Autodesk Fusion 360 part; units mm, degrees
(part 2 of 2)
sketch "Sketch5" plane through (0, 0, 3) normal (0, 0, 1) x (-1, 0, 0)
  circle A0 centre (19.806368, 49.24591) radius 1.5
  circle A1 centre (-47.207036, 20.58349) radius 1.5
  circle A2 centre (47.000001, -22) radius 1.5
  circle A3 centre (-21.042031, -45.95674) radius 1.5
  arc A4 (55, 15) -> (15, 55) centre (15, 15) ccw
  line L0 (15, 55) -> (-15, 55)
  arc A5 (-15, 55) -> (-55, 15) centre (-15, 15) ccw
  line L1 (-55, 15) -> (-55, -15)
  arc A6 (-55, -15) -> (-15, -55) centre (-15, -15) ccw
  line L2 (-15, -55) -> (15, -55)
  arc A7 (15, -55) -> (55, -15) centre (15, -15) ccw
  line L3 (55, -15) -> (55, 15)
  spline S0 degree 3 poles (33.028609, 28.071836) (33.020542, 28.201801) (33.037938, 28.332099) (33.121694, 28.578692) (33.187255, 28.69263) (33.35836, 28.888963) (33.462269, 28.969481) (33.695102, 29.086154) (33.821799, 29.121194) (34.01862, 29.136006) (34.085931, 29.134286) (34.219188, 29.117378) (34.284796, 29.102233) (34.348388, 29.080627) knots 0 0 0 0 0.03906445 0.03906445 0.07812889 0.07812889 0.11719334 0.11719334 0.15625779 0.15625779 0.17640658 0.17640658 0.19655538 0.19655538 0.19655538 0.19655538
  spline S1 degree 3 poles (33.028609, 28.071836) (33.070325, 27.399743) (33.167612, 26.697689) (33.534795, 25.632572) (33.720748, 25.326789) (34.102443, 24.870238) (34.323648, 24.704363) (34.841834, 24.437201) (35.152732, 24.346965) (36.444281, 24.071142) (37.766512, 23.970732) (40.258569, 22.861355) (41.159058, 22.248794) (42.580431, 20.763821) (43.105542, 19.944649) (43.820617, 18.088798) (43.981774, 17.098841) (44.002724, 14.699008) (43.726283, 13.299817) (42.523118, 9.293833) (41.144668, 6.638018) (39.093015, 2.019583) (38.33328, 0.102917) (37.445131, -3.451458) (37.219765, -4.824183) (37.092807, -6.21584) knots 0.12920252 0.12920252 0.12920252 0.12920252 0.29400635 0.29400635 0.41743504 0.41743504 0.55008159 0.55008159 0.70447822 0.70447822 1.12919382 1.12919382 1.40886872 1.40886872 1.66213987 1.66213987 1.92272299 1.92272299 2.28120027 2.28120027 3.00174739 3.00174739 3.49260172 3.49260172 3.80923678 3.80923678 3.80923678 3.80923678
  spline S2 degree 3 poles (38.088834, -7.30669) (37.958619, -7.306711) (37.829645, -7.281298) (37.588698, -7.182465) (37.479028, -7.10999) (37.293642, -6.927081) (37.219699, -6.818395) (37.13638, -6.622803) (37.113583, -6.543309) (37.088005, -6.380538) (37.085323, -6.297883) (37.092807, -6.21584) knots 0 0 0 0 0.03906445 0.03906445 0.07812889 0.07812889 0.11719334 0.11719334 0.14190861 0.14190861 0.16662387 0.16662387 0.16662387 0.16662387
  line L4 (38.088834, -7.30669) -> (44.477012, 2.623123)
  arc A8 (49.249836, -0.9845) -> (44.477012, 2.623123) centre (47.000001, 1) ccw
  line L5 (49.249836, -0.9845) -> (41.439374, -9.839254)
  line L6 (41.439374, -9.839254) -> (37.553028, -14.980826)
  spline S3 degree 3 poles (37.355491, -15.680812) (37.343423, -15.556976) (37.354571, -15.431969) (37.422156, -15.192477) (37.478002, -15.080084) (37.553028, -14.980826) knots 0 0 0 0 0.03732672 0.03732672 0.07465345 0.07465345 0.07465345 0.07465345
  spline S4 degree 3 poles (37.355491, -15.680812) (37.717512, -19.395606) (38.115975, -22.808309) (37.32032, -26.055888) (37.037048, -26.721878) (36.287107, -27.771965) (35.864089, -28.165019) (34.777138, -28.862662) (34.111926, -29.125105) (33.399815, -29.330821) knots 0.03917141 0.03917141 0.03917141 0.03917141 1.16482767 1.16482767 1.51694644 1.51694644 1.81940977 1.81940977 2.17139083 2.17139083 2.17139083 2.17139083
  spline S5 degree 3 poles (32.689476, -30.136274) (32.709693, -30.007638) (32.754843, -29.884181) (32.889924, -29.661523) (32.978563, -29.56445) (33.178711, -29.416652) (33.285884, -29.363733) (33.399815, -29.330821) knots 0 0 0 0 0.03906445 0.03906445 0.07812889 0.07812889 0.11370578 0.11370578 0.11370578 0.11370578
  line L7 (32.689476, -30.136274) -> (31.798898, -35.802654)
  line L8 (31.798898, -35.802654) -> (29.963534, -47.466334)
  arc A9 (24.140467, -46.09277) -> (29.963534, -47.466334) centre (27, -47.000001) ccw
  line L9 (24.140467, -46.09277) -> (27.711083, -34.838407)
  line L10 (27.711083, -34.838407) -> (28.342134, -32.16314)
  spline S6 degree 3 poles (26.916548, -31.04169) (27.032682, -30.982795) (27.15921, -30.947146) (27.418808, -30.926354) (27.549397, -30.94141) (27.797453, -31.020732) (27.912548, -31.084239) (28.111917, -31.251796) (28.194285, -31.354245) (28.310066, -31.575309) (28.346065, -31.690083) (28.375918, -31.926876) (28.369531, -32.046994) (28.342134, -32.16314) knots 0 0 0 0 0.03906445 0.03906445 0.07812889 0.07812889 0.11719334 0.11719334 0.15625779 0.15625779 0.1920579 0.1920579 0.227858 0.227858 0.227858 0.227858
  spline S7 degree 3 poles (26.916548, -31.04169) (26.501678, -31.252085) (26.107211, -31.499509) (24.939768, -32.410184) (24.29803, -33.165919) (22.091994, -36.254574) (20.565282, -39.28296) (15.831093, -43.406948) (14.024745, -44.411258) (11.181859, -45.397232) (9.989834, -45.607) (8.140393, -45.536834) (7.398883, -45.389219) (6.139798, -44.814776) (5.640001, -44.453149) (4.7208, -43.481488) (4.349579, -42.883055) (3.462916, -41.050115) (3.101277, -39.69498) (2.31369, -37.647221) (1.945545, -36.882494) (1.036613, -35.79784) (0.593737, -35.439307) (-0.469029, -34.890024) (-1.078331, -34.709667) (-2.902765, -34.442063) (-4.21808, -34.494421) (-5.659673, -34.662249) knots 0.20837114 0.20837114 0.20837114 0.20837114 0.35937386 0.35937386 0.67047774 0.67047774 1.4465987 1.4465987 1.89541729 1.89541729 2.22492207 2.22492207 2.45047306 2.45047306 2.6397202 2.6397202 2.85015814 2.85015814 3.24794097 3.24794097 3.51947787 3.51947787 3.71561689 3.71561689 3.91564309 3.91564309 4.24291454 4.24291454 4.24291454 4.24291454
  spline S8 degree 3 poles (-6.267359, -36.346049) (-6.357274, -36.251862) (-6.427932, -36.141013) (-6.52278, -35.898469) (-6.546064, -35.769094) (-6.54173, -35.5087) (-6.514153, -35.380172) (-6.411285, -35.140919) (-6.336977, -35.032483) (-6.165307, -34.864241) (-6.074436, -34.800666) (-5.875645, -34.705715) (-5.769085, -34.674986) (-5.659673, -34.662249) knots 0 0 0 0 0.03906445 0.03906445 0.07812889 0.07812889 0.11719334 0.11719334 0.15625779 0.15625779 0.18930324 0.18930324 0.2223487 0.2223487 0.2223487 0.2223487
  line L11 (-6.267359, -36.346049) -> (-5.767132, -36.870049)
  line L12 (-5.767132, -36.870049) -> (3.007378, -44.770554)
  arc A10 (-1.320176, -48.901784) -> (3.007378, -44.770554) centre (1, -47.000001) ccw
  line L13 (-1.320176, -48.901784) -> (-11.749599, -36.177887)
  spline S9 degree 3 poles (-12.684916, -35.825011) (-12.55642, -35.803926) (-12.425033, -35.808141) (-12.191152, -35.862108) (-12.088945, -35.904256) (-11.902341, -36.020074) (-11.819212, -36.092959) (-11.749599, -36.177887) knots 0 0 0 0 0.03906445 0.03906445 0.07200812 0.07200812 0.1049518 0.1049518 0.1049518 0.1049518
  spline S10 degree 3 poles (-12.684916, -35.825011) (-15.152305, -36.229886) (-17.56612, -36.507138) (-20.617728, -36.140773) (-21.595405, -35.894944) (-23.151598, -35.065944) (-23.73315, -34.591978) (-24.687849, -33.42352) (-25.03938, -32.77321) (-25.502185, -31.577004) (-25.653053, -31.047073) (-25.769625, -30.511953) knots 0.05769777 0.05769777 0.05769777 0.05769777 0.81058803 0.81058803 1.16886844 1.16886844 1.44619299 1.44619299 1.71282967 1.71282967 1.90895598 1.90895598 1.90895598 1.90895598
  spline S11 degree 3 poles (-26.760211, -29.724895) (-26.630008, -29.723137) (-26.500707, -29.746827) (-26.258463, -29.842438) (-26.147836, -29.913444) (-25.982773, -30.072013) (-25.922122, -30.150529) (-25.825786, -30.322765) (-25.790628, -30.41554) (-25.769625, -30.511953) knots 0 0 0 0 0.03906445 0.03906445 0.07812889 0.07812889 0.107731 0.107731 0.13733311 0.13733311 0.13733311 0.13733311
  line L14 (-26.760211, -29.724895) -> (-35.15287, -29.83822)
  line L15 (-35.15287, -29.83822) -> (-46.958966, -29.99972)
  arc A11 (-46.588905, -24.0283) -> (-46.958966, -29.99972) centre (-47.000001, -27) ccw
  line L16 (-46.588905, -24.0283) -> (-34.893086, -25.646262)
  line L17 (-34.893086, -25.646262) -> (-27.2325, -26.121004)
  spline S12 degree 3 poles (-26.170767, -25.138463) (-26.172791, -25.268662) (-26.200227, -25.397221) (-26.302832, -25.636586) (-26.377021, -25.745104) (-26.562819, -25.927594) (-26.672653, -25.999821) (-26.862592, -26.077231) (-26.934903, -26.097616) (-27.082715, -26.121857) (-27.15775, -26.125636) (-27.2325, -26.121004) knots 0 0 0 0 0.03906445 0.03906445 0.07812889 0.07812889 0.11719334 0.11719334 0.13966134 0.13966134 0.16212934 0.16212934 0.16212934 0.16212934
  spline S13 degree 3 poles (-26.170767, -25.138463) (-26.10385, -20.833987) (-25.471174, -16.204979) (-26.544717, -7.681658) (-27.73616, -4.599407) (-31.188004, 2.436605) (-33.265635, 6.07333) (-34.771789, 9.827038) knots 0.10413309 0.10413309 0.10413309 0.10413309 1.3791009 1.3791009 2.41617104 2.41617104 3.40624296 3.40624296 3.40624296 3.40624296
  spline S14 degree 3 poles (-36.512881, 10.036897) (-36.437064, 10.142763) (-36.341294, 10.232809) (-36.120628, 10.371122) (-35.997843, 10.418066) (-35.741188, 10.462248) (-35.609773, 10.459062) (-35.35556, 10.402497) (-35.235194, 10.349658) (-35.048762, 10.219811) (-34.977667, 10.153102) (-34.856917, 10.001316) (-34.807902, 9.917042) (-34.771789, 9.827038) knots 0 0 0 0 0.03906445 0.03906445 0.07812889 0.07812889 0.11719334 0.11719334 0.15625779 0.15625779 0.18535143 0.18535143 0.21444508 0.21444508 0.21444508 0.21444508
  line L18 (-36.512881, 10.036897) -> (-38.305738, 7.533451)
  line L19 (-38.305738, 7.533451) -> (-44.436043, -2.557602)
  arc A12 (-49.300203, 0.925894) -> (-44.436043, -2.557602) centre (-47.000001, -1) ccw
  line L20 (-49.300203, 0.925894) -> (-41.720395, 9.978878)
  line L21 (-41.720395, 9.978878) -> (-36.901029, 16.708373)
  spline S15 degree 3 poles (-36.717088, 17.368596) (-36.707973, 17.252065) (-36.71936, 17.134833) (-36.782101, 16.909635) (-36.832972, 16.803404) (-36.901029, 16.708373) knots 0 0 0 0 0.03506615 0.03506615 0.07013231 0.07013231 0.07013231 0.07013231
  spline S16 degree 3 poles (-36.717088, 17.368596) (-36.851793, 19.090796) (-36.725294, 20.800665) (-35.82491, 23.830023) (-35.192711, 25.085877) (-33.574997, 27.33099) (-32.636218, 28.298843) (-31.606983, 29.157724) knots 0.03608701 0.03608701 0.03608701 0.03608701 0.555731 0.555731 0.98365139 0.98365139 1.38609526 1.38609526 1.38609526 1.38609526
  spline S17 degree 3 poles (-31.250302, 29.853272) (-31.259708, 29.723397) (-31.294392, 29.596602) (-31.383142, 29.418243) (-31.420195, 29.359812) (-31.50574, 29.251513) (-31.554002, 29.201936) (-31.606983, 29.157724) knots 0 0 0 0 0.03906445 0.03906445 0.05976579 0.05976579 0.08046713 0.08046713 0.08046713 0.08046713
  line L22 (-31.250302, 29.853272) -> (-30.845628, 35.440539)
  line L23 (-30.845628, 35.440539) -> (-29.992153, 47.216854)
  arc A13 (-24.074611, 46.335098) -> (-29.992153, 47.216854) centre (-27, 47.000001) ccw
  line L24 (-24.074611, 46.335098) -> (-26.691493, 34.821543)
  line L25 (-26.691493, 34.821543) -> (-26.827892, 33.906158)
  spline S18 degree 3 poles (-25.443022, 32.840437) (-25.562603, 32.788899) (-25.691108, 32.761211) (-25.951498, 32.756651) (-26.080893, 32.779823) (-26.323519, 32.874462) (-26.434429, 32.945024) (-26.62296, 33.12469) (-26.698777, 33.232076) (-26.790548, 33.437548) (-26.816707, 33.529187) (-26.842431, 33.717075) (-26.841866, 33.812373) (-26.827892, 33.906158) knots 0 0 0 0 0.03906445 0.03906445 0.07812889 0.07812889 0.11719334 0.11719334 0.15625779 0.15625779 0.1847039 0.1847039 0.21315002 0.21315002 0.21315002 0.21315002
  spline S19 degree 3 poles (-25.443022, 32.840437) (-22.639111, 34.048877) (-19.64058, 34.864689) (-13.990802, 35.609538) (-11.903288, 35.347809) (-8.639296, 34.492873) (-7.24095, 33.736993) (-4.677922, 32.21498) (-3.539006, 31.471178) (-1.766627, 30.825805) (-1.13553, 30.690347) (0.120331, 30.722159) (0.684409, 30.86072) (1.959514, 31.399025) (2.667406, 31.871418) (4.176502, 33.086706) (4.982409, 33.852701) (5.832592, 34.675606) knots 0.18219729 0.18219729 0.18219729 0.18219729 1.09067944 1.09067944 2.11663156 2.11663156 3.31549349 3.31549349 4.45967423 4.45967423 5.07162521 5.07162521 5.62607132 5.62607132 6.35980303 6.35980303 7.15795757 7.15795757 7.15795757 7.15795757
  spline S20 degree 3 poles (5.885742, 36.057127) (5.972072, 35.959644) (6.038536, 35.84623) (6.124249, 35.600309) (6.142679, 35.470154) (6.128612, 35.210105) (6.096249, 35.082697) (5.989005, 34.856928) (5.918623, 34.758878) (5.832592, 34.675606) knots 0 0 0 0 0.03906445 0.03906445 0.07812889 0.07812889 0.11719334 0.11719334 0.15311273 0.15311273 0.15311273 0.15311273
  line L26 (5.885742, 36.057127) -> (5.383635, 36.624105)
  line L27 (5.383635, 36.624105) -> (-3.089335, 44.84717)
  arc A14 (1.389663, 48.813702) -> (-3.089335, 44.84717) centre (-1, 47.000001) ccw
  line L28 (1.389663, 48.813702) -> (8.527907, 39.408625)
  line L29 (8.527907, 39.408625) -> (8.997232, 38.878665)
  spline S21 degree 3 poles (10.353438, 38.74738) (10.250013, 38.668265) (10.132124, 38.610108) (9.880688, 38.542257) (9.749546, 38.53321) (9.500962, 38.564658) (9.385265, 38.601194) (9.172426, 38.713607) (9.077022, 38.788566) (8.997232, 38.878665) knots 0 0 0 0 0.03906445 0.03906445 0.07812889 0.07812889 0.11423407 0.11423407 0.15033925 0.15033925 0.15033925 0.15033925
  spline S22 degree 3 poles (10.353438, 38.74738) (11.733539, 39.803082) (13.210331, 40.705104) (16.432276, 41.90028) (18.061322, 42.165253) (21.42658, 42.026481) (23.073064, 41.629511) (26.565289, 40.202857) (28.314525, 39.054702) (30.298495, 37.237861) (30.878286, 36.616261) (31.702413, 35.507726) (32.000821, 35.03614) (32.246808, 34.538749) knots 0.09311255 0.09311255 0.09311255 0.09311255 0.61605828 0.61605828 1.12703458 1.12703458 1.63347766 1.63347766 2.26940705 2.26940705 2.55315447 2.55315447 2.74216348 2.74216348 2.74216348 2.74216348
  spline S23 degree 3 poles (32.821479, 34.035211) (32.698186, 34.077101) (32.584254, 34.142673) (32.38663, 34.314936) (32.305301, 34.420473) (32.246808, 34.538749) knots 0 0 0 0 0.03906445 0.03906445 0.07864923 0.07864923 0.07864923 0.07864923
  line L30 (32.821479, 34.035211) -> (36.313471, 32.848768)
  line L31 (36.313471, 32.848768) -> (47.747888, 29.90528)
  arc A15 (45.823197, 24.240447) -> (47.747889, 29.905282) centre (47.000001, 27) ccw
  line L32 (45.823197, 24.240447) -> (34.962331, 28.872033)
  line L33 (34.962331, 28.872033) -> (34.348388, 29.080627)
  circle A16 centre (-14, 47.000001) radius 1.5
  circle A17 centre (47.000001, 14) radius 1.5
  circle A18 centre (-47.000001, -14) radius 1.5
  circle A19 centre (14, -47.000001) radius 1.5
  circle A20 centre (-38.15, -37.75) radius 2.75
  circle A21 centre (37.75, -38.15) radius 2.75
  circle A22 centre (-37.75, 38.15) radius 2.75
  circle A23 centre (38.15, 37.75) radius 2.75
  circle A24 centre (19.806368, 49.24591) radius 4
  line L34 (15.806368, 49.24591) -> (15.806368, 54.991871)
  line L35 (23.806368, 49.24591) -> (23.806368, 54.018558)
  dimension "d135" = 8
  constraint concentric A0 A24
  constraint tangent A24 L34
  constraint vertical L34
  constraint tangent A24 L35
  constraint parallel L34 L35
  measures "d135" diameter of A24
sketch "LaserMidPlateShell" plane through (0, 0, 3) normal (0, 0, 1) x (-1, 0, 0)
  circle A0 centre (19.806368, 49.24591) radius 1.5
  circle A1 centre (-47.207036, 20.58349) radius 1.5
  circle A2 centre (47.000001, -22) radius 1.5
  circle A3 centre (-21.042031, -45.95674) radius 1.5
  arc A4 (55, 15) -> (15, 55) centre (15, 15) ccw
  line L0 (15, 55) -> (-15, 55)
  arc A5 (-15, 55) -> (-55, 15) centre (-15, 15) ccw
  line L1 (-55, 15) -> (-55, -15)
  arc A6 (-55, -15) -> (-15, -55) centre (-15, -15) ccw
  line L2 (-15, -55) -> (15, -55)
  arc A7 (15, -55) -> (55, -15) centre (15, -15) ccw
  line L3 (55, -15) -> (55, 15)
  spline S0 degree 3 poles (33.028609, 28.071836) (33.020542, 28.201801) (33.037938, 28.332099) (33.121694, 28.578692) (33.187255, 28.69263) (33.35836, 28.888963) (33.462269, 28.969481) (33.695102, 29.086154) (33.821799, 29.121194) (34.01862, 29.136006) (34.085931, 29.134286) (34.219188, 29.117378) (34.284796, 29.102233) (34.348388, 29.080627) knots 0 0 0 0 0.03906445 0.03906445 0.07812889 0.07812889 0.11719334 0.11719334 0.15625779 0.15625779 0.17640658 0.17640658 0.19655538 0.19655538 0.19655538 0.19655538
  spline S1 degree 3 poles (33.028609, 28.071836) (33.070325, 27.399743) (33.167612, 26.697689) (33.534795, 25.632572) (33.720748, 25.326789) (34.102443, 24.870238) (34.323648, 24.704363) (34.841834, 24.437201) (35.152732, 24.346965) (36.444281, 24.071142) (37.766512, 23.970732) (40.258569, 22.861355) (41.159058, 22.248794) (42.580431, 20.763821) (43.105542, 19.944649) (43.820617, 18.088798) (43.981774, 17.098841) (44.002724, 14.699008) (43.726283, 13.299817) (42.523118, 9.293833) (41.144668, 6.638018) (39.093015, 2.019583) (38.33328, 0.102917) (37.445131, -3.451458) (37.219765, -4.824183) (37.092807, -6.21584) knots 0.12920252 0.12920252 0.12920252 0.12920252 0.29400635 0.29400635 0.41743504 0.41743504 0.55008159 0.55008159 0.70447822 0.70447822 1.12919382 1.12919382 1.40886872 1.40886872 1.66213987 1.66213987 1.92272299 1.92272299 2.28120027 2.28120027 3.00174739 3.00174739 3.49260172 3.49260172 3.80923678 3.80923678 3.80923678 3.80923678
  spline S2 degree 3 poles (38.088834, -7.30669) (37.958619, -7.306711) (37.829645, -7.281298) (37.588698, -7.182465) (37.479028, -7.10999) (37.293642, -6.927081) (37.219699, -6.818395) (37.13638, -6.622803) (37.113583, -6.543309) (37.088005, -6.380538) (37.085323, -6.297883) (37.092807, -6.21584) knots 0 0 0 0 0.03906445 0.03906445 0.07812889 0.07812889 0.11719334 0.11719334 0.14190861 0.14190861 0.16662387 0.16662387 0.16662387 0.16662387
  line L4 (38.088834, -7.30669) -> (44.477012, 2.623123)
  arc A8 (49.249836, -0.9845) -> (44.477012, 2.623123) centre (47.000001, 1) ccw
  line L5 (49.249836, -0.9845) -> (41.439374, -9.839254)
  line L6 (41.439374, -9.839254) -> (37.553028, -14.980826)
  spline S3 degree 3 poles (37.355491, -15.680812) (37.343423, -15.556976) (37.354571, -15.431969) (37.422156, -15.192477) (37.478002, -15.080084) (37.553028, -14.980826) knots 0 0 0 0 0.03732672 0.03732672 0.07465345 0.07465345 0.07465345 0.07465345
  spline S4 degree 3 poles (37.355491, -15.680812) (37.717512, -19.395606) (38.115975, -22.808309) (37.32032, -26.055888) (37.037048, -26.721878) (36.287107, -27.771965) (35.864089, -28.165019) (34.777138, -28.862662) (34.111926, -29.125105) (33.399815, -29.330821) knots 0.03917141 0.03917141 0.03917141 0.03917141 1.16482767 1.16482767 1.51694644 1.51694644 1.81940977 1.81940977 2.17139083 2.17139083 2.17139083 2.17139083
  spline S5 degree 3 poles (32.689476, -30.136274) (32.709693, -30.007638) (32.754843, -29.884181) (32.889924, -29.661523) (32.978563, -29.56445) (33.178711, -29.416652) (33.285884, -29.363733) (33.399815, -29.330821) knots 0 0 0 0 0.03906445 0.03906445 0.07812889 0.07812889 0.11370578 0.11370578 0.11370578 0.11370578
  line L7 (32.689476, -30.136274) -> (31.798898, -35.802654)
  line L8 (31.798898, -35.802654) -> (29.963534, -47.466334)
  arc A9 (24.140467, -46.09277) -> (29.963534, -47.466334) centre (27, -47.000001) ccw
  line L9 (24.140467, -46.09277) -> (27.711083, -34.838407)
  line L10 (27.711083, -34.838407) -> (28.342134, -32.16314)
  spline S6 degree 3 poles (26.916548, -31.04169) (27.032682, -30.982795) (27.15921, -30.947146) (27.418808, -30.926354) (27.549397, -30.94141) (27.797453, -31.020732) (27.912548, -31.084239) (28.111917, -31.251796) (28.194285, -31.354245) (28.310066, -31.575309) (28.346065, -31.690083) (28.375918, -31.926876) (28.369531, -32.046994) (28.342134, -32.16314) knots 0 0 0 0 0.03906445 0.03906445 0.07812889 0.07812889 0.11719334 0.11719334 0.15625779 0.15625779 0.1920579 0.1920579 0.227858 0.227858 0.227858 0.227858
  spline S7 degree 3 poles (26.916548, -31.04169) (26.501678, -31.252085) (26.107211, -31.499509) (24.939768, -32.410184) (24.29803, -33.165919) (22.091994, -36.254574) (20.565282, -39.28296) (15.831093, -43.406948) (14.024745, -44.411258) (11.181859, -45.397232) (9.989834, -45.607) (8.140393, -45.536834) (7.398883, -45.389219) (6.139798, -44.814776) (5.640001, -44.453149) (4.7208, -43.481488) (4.349579, -42.883055) (3.462916, -41.050115) (3.101277, -39.69498) (2.31369, -37.647221) (1.945545, -36.882494) (1.036613, -35.79784) (0.593737, -35.439307) (-0.469029, -34.890024) (-1.078331, -34.709667) (-2.902765, -34.442063) (-4.21808, -34.494421) (-5.659673, -34.662249) knots 0.20837114 0.20837114 0.20837114 0.20837114 0.35937386 0.35937386 0.67047774 0.67047774 1.4465987 1.4465987 1.89541729 1.89541729 2.22492207 2.22492207 2.45047306 2.45047306 2.6397202 2.6397202 2.85015814 2.85015814 3.24794097 3.24794097 3.51947787 3.51947787 3.71561689 3.71561689 3.91564309 3.91564309 4.24291454 4.24291454 4.24291454 4.24291454
  spline S8 degree 3 poles (-6.267359, -36.346049) (-6.357274, -36.251862) (-6.427932, -36.141013) (-6.52278, -35.898469) (-6.546064, -35.769094) (-6.54173, -35.5087) (-6.514153, -35.380172) (-6.411285, -35.140919) (-6.336977, -35.032483) (-6.165307, -34.864241) (-6.074436, -34.800666) (-5.875645, -34.705715) (-5.769085, -34.674986) (-5.659673, -34.662249) knots 0 0 0 0 0.03906445 0.03906445 0.07812889 0.07812889 0.11719334 0.11719334 0.15625779 0.15625779 0.18930324 0.18930324 0.2223487 0.2223487 0.2223487 0.2223487
  line L11 (-6.267359, -36.346049) -> (-5.767132, -36.870049)
  line L12 (-5.767132, -36.870049) -> (3.007378, -44.770554)
  arc A10 (-1.320176, -48.901784) -> (3.007378, -44.770554) centre (1, -47.000001) ccw
  line L13 (-1.320176, -48.901784) -> (-11.749599, -36.177887)
  spline S9 degree 3 poles (-12.684916, -35.825011) (-12.55642, -35.803926) (-12.425033, -35.808141) (-12.191152, -35.862108) (-12.088945, -35.904256) (-11.902341, -36.020074) (-11.819212, -36.092959) (-11.749599, -36.177887) knots 0 0 0 0 0.03906445 0.03906445 0.07200812 0.07200812 0.1049518 0.1049518 0.1049518 0.1049518
  spline S10 degree 3 poles (-12.684916, -35.825011) (-15.152305, -36.229886) (-17.56612, -36.507138) (-20.617728, -36.140773) (-21.595405, -35.894944) (-23.151598, -35.065944) (-23.73315, -34.591978) (-24.687849, -33.42352) (-25.03938, -32.77321) (-25.502185, -31.577004) (-25.653053, -31.047073) (-25.769625, -30.511953) knots 0.05769777 0.05769777 0.05769777 0.05769777 0.81058803 0.81058803 1.16886844 1.16886844 1.44619299 1.44619299 1.71282967 1.71282967 1.90895598 1.90895598 1.90895598 1.90895598
  spline S11 degree 3 poles (-26.760211, -29.724895) (-26.630008, -29.723137) (-26.500707, -29.746827) (-26.258463, -29.842438) (-26.147836, -29.913444) (-25.982773, -30.072013) (-25.922122, -30.150529) (-25.825786, -30.322765) (-25.790628, -30.41554) (-25.769625, -30.511953) knots 0 0 0 0 0.03906445 0.03906445 0.07812889 0.07812889 0.107731 0.107731 0.13733311 0.13733311 0.13733311 0.13733311
  line L14 (-26.760211, -29.724895) -> (-35.15287, -29.83822)
  line L15 (-35.15287, -29.83822) -> (-46.958966, -29.99972)
  arc A11 (-46.588905, -24.0283) -> (-46.958966, -29.99972) centre (-47.000001, -27) ccw
  line L16 (-46.588905, -24.0283) -> (-34.893086, -25.646262)
  line L17 (-34.893086, -25.646262) -> (-27.2325, -26.121004)
  spline S12 degree 3 poles (-26.170767, -25.138463) (-26.172791, -25.268662) (-26.200227, -25.397221) (-26.302832, -25.636586) (-26.377021, -25.745104) (-26.562819, -25.927594) (-26.672653, -25.999821) (-26.862592, -26.077231) (-26.934903, -26.097616) (-27.082715, -26.121857) (-27.15775, -26.125636) (-27.2325, -26.121004) knots 0 0 0 0 0.03906445 0.03906445 0.07812889 0.07812889 0.11719334 0.11719334 0.13966134 0.13966134 0.16212934 0.16212934 0.16212934 0.16212934
  spline S13 degree 3 poles (-26.170767, -25.138463) (-26.10385, -20.833987) (-25.471174, -16.204979) (-26.544717, -7.681658) (-27.73616, -4.599407) (-31.188004, 2.436605) (-33.265635, 6.07333) (-34.771789, 9.827038) knots 0.10413309 0.10413309 0.10413309 0.10413309 1.3791009 1.3791009 2.41617104 2.41617104 3.40624296 3.40624296 3.40624296 3.40624296
  spline S14 degree 3 poles (-36.512881, 10.036897) (-36.437064, 10.142763) (-36.341294, 10.232809) (-36.120628, 10.371122) (-35.997843, 10.418066) (-35.741188, 10.462248) (-35.609773, 10.459062) (-35.35556, 10.402497) (-35.235194, 10.349658) (-35.048762, 10.219811) (-34.977667, 10.153102) (-34.856917, 10.001316) (-34.807902, 9.917042) (-34.771789, 9.827038) knots 0 0 0 0 0.03906445 0.03906445 0.07812889 0.07812889 0.11719334 0.11719334 0.15625779 0.15625779 0.18535143 0.18535143 0.21444508 0.21444508 0.21444508 0.21444508
  line L18 (-36.512881, 10.036897) -> (-38.305738, 7.533451)
  line L19 (-38.305738, 7.533451) -> (-44.436043, -2.557602)
  arc A12 (-49.300203, 0.925894) -> (-44.436043, -2.557602) centre (-47.000001, -1) ccw
  line L20 (-49.300203, 0.925894) -> (-41.720395, 9.978878)
  line L21 (-41.720395, 9.978878) -> (-36.901029, 16.708373)
  spline S15 degree 3 poles (-36.717088, 17.368596) (-36.707973, 17.252065) (-36.71936, 17.134833) (-36.782101, 16.909635) (-36.832972, 16.803404) (-36.901029, 16.708373) knots 0 0 0 0 0.03506615 0.03506615 0.07013231 0.07013231 0.07013231 0.07013231
  spline S16 degree 3 poles (-36.717088, 17.368596) (-36.851793, 19.090796) (-36.725294, 20.800665) (-35.82491, 23.830023) (-35.192711, 25.085877) (-33.574997, 27.33099) (-32.636218, 28.298843) (-31.606983, 29.157724) knots 0.03608701 0.03608701 0.03608701 0.03608701 0.555731 0.555731 0.98365139 0.98365139 1.38609526 1.38609526 1.38609526 1.38609526
  spline S17 degree 3 poles (-31.250302, 29.853272) (-31.259708, 29.723397) (-31.294392, 29.596602) (-31.383142, 29.418243) (-31.420195, 29.359812) (-31.50574, 29.251513) (-31.554002, 29.201936) (-31.606983, 29.157724) knots 0 0 0 0 0.03906445 0.03906445 0.05976579 0.05976579 0.08046713 0.08046713 0.08046713 0.08046713
  line L22 (-31.250302, 29.853272) -> (-30.845628, 35.440539)
  line L23 (-30.845628, 35.440539) -> (-29.992153, 47.216854)
  arc A13 (-24.074611, 46.335098) -> (-29.992153, 47.216854) centre (-27, 47.000001) ccw
  line L24 (-24.074611, 46.335098) -> (-26.691493, 34.821543)
  line L25 (-26.691493, 34.821543) -> (-26.827892, 33.906158)
  spline S18 degree 3 poles (-25.443022, 32.840437) (-25.562603, 32.788899) (-25.691108, 32.761211) (-25.951498, 32.756651) (-26.080893, 32.779823) (-26.323519, 32.874462) (-26.434429, 32.945024) (-26.62296, 33.12469) (-26.698777, 33.232076) (-26.790548, 33.437548) (-26.816707, 33.529187) (-26.842431, 33.717075) (-26.841866, 33.812373) (-26.827892, 33.906158) knots 0 0 0 0 0.03906445 0.03906445 0.07812889 0.07812889 0.11719334 0.11719334 0.15625779 0.15625779 0.1847039 0.1847039 0.21315002 0.21315002 0.21315002 0.21315002
  spline S19 degree 3 poles (-25.443022, 32.840437) (-22.639111, 34.048877) (-19.64058, 34.864689) (-13.990802, 35.609538) (-11.903288, 35.347809) (-8.639296, 34.492873) (-7.24095, 33.736993) (-4.677922, 32.21498) (-3.539006, 31.471178) (-1.766627, 30.825805) (-1.13553, 30.690347) (0.120331, 30.722159) (0.684409, 30.86072) (1.959514, 31.399025) (2.667406, 31.871418) (4.176502, 33.086706) (4.982409, 33.852701) (5.832592, 34.675606) knots 0.18219729 0.18219729 0.18219729 0.18219729 1.09067944 1.09067944 2.11663156 2.11663156 3.31549349 3.31549349 4.45967423 4.45967423 5.07162521 5.07162521 5.62607132 5.62607132 6.35980303 6.35980303 7.15795757 7.15795757 7.15795757 7.15795757
  spline S20 degree 3 poles (5.885742, 36.057127) (5.972072, 35.959644) (6.038536, 35.84623) (6.124249, 35.600309) (6.142679, 35.470154) (6.128612, 35.210105) (6.096249, 35.082697) (5.989005, 34.856928) (5.918623, 34.758878) (5.832592, 34.675606) knots 0 0 0 0 0.03906445 0.03906445 0.07812889 0.07812889 0.11719334 0.11719334 0.15311273 0.15311273 0.15311273 0.15311273
  line L26 (5.885742, 36.057127) -> (5.383635, 36.624105)
  line L27 (5.383635, 36.624105) -> (-3.089335, 44.84717)
  arc A14 (1.389663, 48.813702) -> (-3.089335, 44.84717) centre (-1, 47.000001) ccw
  line L28 (1.389663, 48.813702) -> (8.527907, 39.408625)
  line L29 (8.527907, 39.408625) -> (8.997232, 38.878665)
  spline S21 degree 3 poles (10.353438, 38.74738) (10.250013, 38.668265) (10.132124, 38.610108) (9.880688, 38.542257) (9.749546, 38.53321) (9.500962, 38.564658) (9.385265, 38.601194) (9.172426, 38.713607) (9.077022, 38.788566) (8.997232, 38.878665) knots 0 0 0 0 0.03906445 0.03906445 0.07812889 0.07812889 0.11423407 0.11423407 0.15033925 0.15033925 0.15033925 0.15033925
  spline S22 degree 3 poles (10.353438, 38.74738) (11.733539, 39.803082) (13.210331, 40.705104) (16.432276, 41.90028) (18.061322, 42.165253) (21.42658, 42.026481) (23.073064, 41.629511) (26.565289, 40.202857) (28.314525, 39.054702) (30.298495, 37.237861) (30.878286, 36.616261) (31.702413, 35.507726) (32.000821, 35.03614) (32.246808, 34.538749) knots 0.09311255 0.09311255 0.09311255 0.09311255 0.61605828 0.61605828 1.12703458 1.12703458 1.63347766 1.63347766 2.26940705 2.26940705 2.55315447 2.55315447 2.74216348 2.74216348 2.74216348 2.74216348
  spline S23 degree 3 poles (32.821479, 34.035211) (32.698186, 34.077101) (32.584254, 34.142673) (32.38663, 34.314936) (32.305301, 34.420473) (32.246808, 34.538749) knots 0 0 0 0 0.03906445 0.03906445 0.07864923 0.07864923 0.07864923 0.07864923
  line L30 (32.821479, 34.035211) -> (36.313471, 32.848768)
  line L31 (36.313471, 32.848768) -> (47.747888, 29.90528)
  arc A15 (45.823197, 24.240447) -> (47.747889, 29.905282) centre (47.000001, 27) ccw
  line L32 (45.823197, 24.240447) -> (34.962331, 28.872033)
  line L33 (34.962331, 28.872033) -> (34.348388, 29.080627)
  circle A16 centre (-14, 47.000001) radius 1.5
  circle A17 centre (47.000001, 14) radius 1.5
  circle A18 centre (-47.000001, -14) radius 1.5
  circle A19 centre (14, -47.000001) radius 1.5
  circle A20 centre (-38.15, -37.75) radius 2.75
  circle A21 centre (37.75, -38.15) radius 2.75
  circle A22 centre (-37.75, 38.15) radius 2.75
  circle A23 centre (38.15, 37.75) radius 2.75
